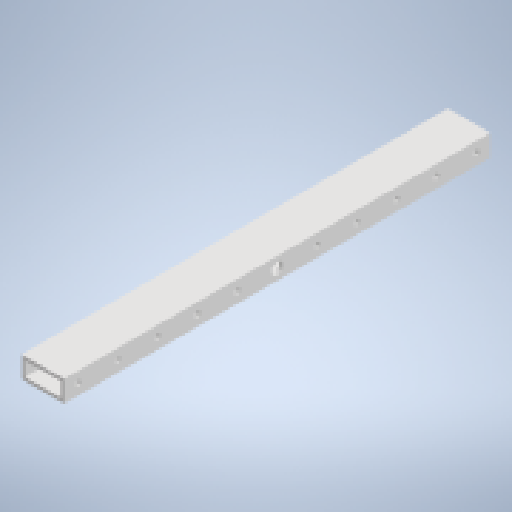
# Autodesk Inventor part: hinge aray side
Saved by Autodesk Inventor 2025.2 (Build 292293000, 293)
## iProperties
Created: 2025-01-08
Part Number: hinge aray side
Material: Generic
Document SubType Name: Modeling
Designer: 5013908
Density: 1 g/cm^3
Appearance: Default
Author: 5013908
Autodesk Inventor part; units mm, degrees
ref_plane "YZ Plane" through (0, 0, 0) normal (1, 0, 0) x (0, 1, 0)
ref_plane "XZ Plane" through (0, 0, 0) normal (0, 1, 0) x (-1, 0, 0)
ref_plane "XY Plane" through (0, 0, 0) normal (0, 0, 1) x (1, 0, 0)
sketch "Sketch1" plane through (0, 0, 0) normal (0, 0, 1) x (1, 0, 0)
  line L0 (0, 0) -> (38.1, 0)
  line L1 (38.1, 0) -> (38.1, 19.05)
  line L2 (38.1, 19.05) -> (0, 19.05)
  line L3 (0, 19.05) -> (0, 0)
  line L4 (3.175, 15.875) -> (34.925, 15.875)
  line L5 (34.925, 15.875) -> (34.925, 3.175)
  line L6 (34.925, 3.175) -> (3.175, 3.175)
  line L7 (3.175, 3.175) -> (3.175, 15.875)
  dimension "d0" = 38.1
  dimension "d1" = 19.05
  dimension "d2" = 3.175
  constraints: 16 end point, 4 parallel, 2 perpendicular, 1 horizontal, 3 other
  measures "d0" distance of L2.end L1.end
  measures "d1" distance of L1.end L0.end
  measures "d2" distance between parallel lines of L2 L4
extrude "Extrusion1" add sketch "Sketch1" along normal blind 381
sketch "Sketch2" plane through (38.1, 0, 0) normal (1, 0, 0) x (0, 0, -1)
  circle A0 centre (-190.5, 9.525) radius 5
  line L0 (0, 19.05) -> (-381, 19.05) projected
  line L1 (-381, 0) -> (-381, 19.05) projected
  point P0 (0, 0)
  point P1 (-381, 9.525)
  dimension "d5" = 10
  dimension "d6" = 9.525
  dimension "d7" = 190.5
  constraints: 1 centre point, 1 midpoint
  measures "d5" diameter of A0
  measures "d6" distance from line of L0 A0.centre
  measures "d7" distance of point (-381, 9.525) A0.centre
extrude "Extrusion2" cut sketch "Sketch2" against normal blind 381
sketch "Sketch4" plane through (38.1, 0, 0) normal (1, 0, 0) x (0, 0, -1)
  line L0 (-381, 0) -> (-381, 19.05) projected
  line L1 (-381, 9.525) -> (-254, 9.525)
  circle A0 centre (-368.3, 9.525) radius 2.5
  circle A1 centre (-332.74, 9.525) radius 2.5
  circle A2 centre (-297.18, 9.525) radius 2.5
  circle A3 centre (-261.62, 9.525) radius 2.5
  circle A4 centre (-226.06, 9.525) radius 2.5
  line L2 (0, 0) -> (0, 19.05) projected
  line L3 (0, 9.525) -> (-40.9904, 9.525)
  circle A5 centre (-12.7, 9.525) radius 2.5
  circle A6 centre (-48.26, 9.525) radius 2.5
  circle A7 centre (-83.82, 9.525) radius 2.5
  circle A8 centre (-119.38, 9.525) radius 2.5
  circle A9 centre (-154.94, 9.525) radius 2.5
  dimension "d10" = 127
  dimension "d11" = 5
  dimension "d14" = 35.56
  dimension "d19" = 12.7
  dimension "d20" = 5
  dimension "d23" = 35.56
  dimension "d28" = 12.7
  constraints: 10 centre point, 4 end point, 4 horizontal, 2 midpoint, 2 point on line, 16 other
  measures "d10" distance of L1.start L1.end
  measures "d11" diameter of A0
  measures "d14" distance of A0.centre A1.centre
  measures "d19" distance from line of L0 A0.centre
  measures "d20" diameter of A5
  measures "d23" distance of A5.centre A6.centre
  measures "d28" distance from line of L2 A5.centre
extrude "Extrusion3" cut sketch "Sketch4" against normal blind 381
body "Solid1"
